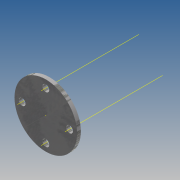
# Autodesk Inventor part: vakkarima2
Saved by Autodesk Inventor 2016 (Build 200138000, 138)
## iProperties
Created: 2017-10-14
Part Number: vakkarima2
Material: Steel, Alloy
Document SubType Name: Modeling
Designer: Fauszt
Density: 7.73 g/cm^3
Appearance: Semi-Polished
Mass: 1574.18 g
Surface Area: 481.748 cm^2
Volume: 203.646 cm^3
Author: Fauszt
Autodesk Inventor part; units mm, degrees
ref_plane "YZ Plane" through (0, 0, 0) normal (1, 0, 0) x (0, 1, 0)
ref_plane "XZ Plane" through (0, 0, 0) normal (0, 1, 0) x (-1, 0, 0)
ref_plane "XY Plane" through (0, 0, 0) normal (0, 0, 1) x (1, 0, 0)
sketch "Sketch1" plane through (0, 0, 0) normal (0, 0, 1) x (1, 0, 0)
  line L0 (-82.5, 3) -> (-82.5, 18) construction
  line L1 (82.5, 3) -> (-82.5, 3) construction
  line L2 (-51, 0) -> (-51, 3) construction
  line L3 (-82.5, 0) -> (-82.5, -10)
  line L4 (-82.5, -10) -> (0, -10)
  line L5 (0, -10) -> (0, 0)
  line L6 (0, 0) -> (-82.5, 0)
  dimension "d0" = 10
  constraints: 12 end point, 3 perpendicular, 3 vertical, 1 point on line, 4 other
  measures "d0" distance of L4.end L5.end
revolve "Revolution1" add sketch "Sketch1" angle 360 about axis through (0, -10, 0) along (0, 1, 0)
sketch "Sketch2" plane through (0, -10, 0) normal (0, -1, 0) x (1, 0, 0)
  circle A0 centre (0, 0) radius 49.3853 construction
  circle A1 centre (-62.5, 0) radius 9.2 projected
  circle A2 centre (0, 62.5) radius 9.2 projected
  circle A3 centre (0, 0) radius 82.3 projected
  circle A4 centre (62.5, 0) radius 9.2 projected
  circle A5 centre (0, -62.5) radius 9.2 projected
  point P0 (0, 0)
  point P1 (62.5, 0)
hole "Hole1" at (62.5, -10, 0) direction (0, 1, 0) diameter 18 end through all
pattern_circular "Circular Pattern1" count 4 over 360 about axis through (0, -10, 0) along (0, 1, 0) of "Hole1"
body "Solid1"
